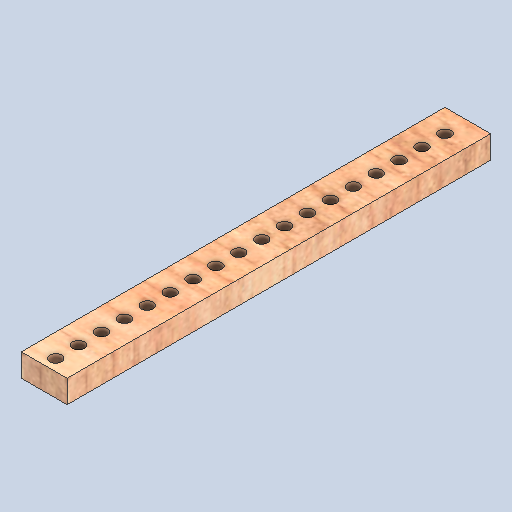
# Autodesk Inventor part: Zarm
Saved by Autodesk Inventor 2023 (Build 270158000, 158)
## iProperties
Created: 2023-10-26
Part Number: Zarm
Material: Wood (Birch)
Document SubType Name: Modeling
Designer: Mustapha
Density: 0.55 g/cm^3
Appearance: Birch - Natural Polished
Mass: 18.2475 g
Surface Area: 136.76 cm^2
Volume: 33.1773 cm^3
Author: Mustapha
Autodesk Inventor part; units mm, degrees
ref_plane "YZ Plane" through (0, 0, 0) normal (1, 0, 0) x (0, 1, 0)
ref_plane "XZ Plane" through (0, 0, 0) normal (0, 1, 0) x (-1, 0, 0)
ref_plane "XY Plane" through (0, 0, 0) normal (0, 0, 1) x (1, 0, 0)
sketch "Sketch1" plane through (0, 0, 0) normal (0, 1, 0) x (-1, 0, 0)
  line L0 (-10, 92.5) -> (10, 92.5)
  line L1 (10, 92.5) -> (10, -92.5)
  line L2 (10, -92.5) -> (-10, -92.5)
  line L3 (-10, -92.5) -> (-10, 92.5)
  line L4 (-10, 92.5) -> (10, -92.5) construction
  line L5 (10, 92.5) -> (-10, -92.5) construction
  circle A0 centre (0, -82.5) radius 2.6
  circle A1 centre (0, -72.5) radius 2.6
  circle A2 centre (0, -62.5) radius 2.6
  circle A3 centre (0, -52.5) radius 2.6
  circle A4 centre (0, -42.5) radius 2.6
  circle A5 centre (0, -32.5) radius 2.6
  circle A6 centre (0, -22.5) radius 2.6
  circle A7 centre (0, -12.5) radius 2.6
  circle A8 centre (0, -2.5) radius 2.6
  circle A9 centre (0, 7.5) radius 2.6
  circle A10 centre (0, 17.5) radius 2.6
  circle A11 centre (0, 27.5) radius 2.6
  circle A12 centre (0, 37.5) radius 2.6
  circle A13 centre (0, 47.5) radius 2.6
  circle A14 centre (0, 57.5) radius 2.6
  circle A15 centre (0, 67.5) radius 2.6
  circle A16 centre (0, 77.5) radius 2.6
  circle A17 centre (0, 87.5) radius 2.6
  circle A18 centre (0, 97.5) radius 2.6
  circle A19 centre (0, 107.5) radius 2.6
  circle A20 centre (0, 117.5) radius 2.6
  circle A21 centre (0, 127.5) radius 2.6
  circle A22 centre (0, 137.5) radius 2.6
  circle A23 centre (0, 147.5) radius 2.6
  point P0 (0, 0)
  dimension "d0" = 20
  dimension "d1" = 185
  dimension "d2" = 10
  dimension "d3" = 5.2
  dimension "d6" = 10
  constraints: 24 centre point, 12 end point, 2 midpoint, 2 parallel, 1 horizontal, 1 perpendicular, 1 vertical, 46 other
  measures "d0" distance between parallel lines of L3 L1
  measures "d1" distance between parallel lines of L0 L2
  measures "d2" distance from line of L2 A0.centre
  measures "d3" diameter of A0
  measures "d6" distance of A0.centre A1.centre
extrude "Extrusion1" add sketch "Sketch1" along normal blind 10 contours L0 L1 L2 L3
body "Solid1"
